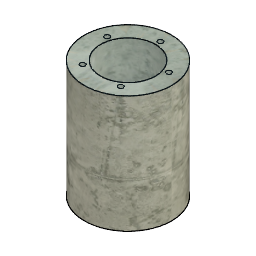
poken door (Autodesk Fusion 360 design; units mm, degrees)
Autodesk Fusion 360 part; units mm, degrees
note: some values were not read from the file. Chosen so that the rebuilt part matches the saved one: where a step ends.
sketch "Esboço1" plane through (0, 0, 0) normal (0, 0, 1) x (1, 0, 0)
  circle A0 centre (0, 0) radius 150
  dimension "d1" = 300
  constraint coincident A0.centre origin
  measures "d1" diameter of A0
extrude "Extrusão1" add sketch "Esboço1" along normal blind 470
sketch "Esboço2" plane through (0, 0, 470) normal (0, 0, 1) x (-1, 0, 0)
  circle A0 centre (0, 0) radius 150
  circle A1 centre (0, 0) radius 175
  dimension "d4" = 350
  constraint coincident A0.centre A1.centre
  measures "d4" diameter of A1
sketch "Esboço3" plane through (0, 0, 470) normal (0, 0, 1) x (-1, 0, 0)
extrude "Extrusão2" add sketch "Esboço2" along normal blind 0 and the other way blind 470
sketch "Esboço4" plane through (0, 0, 470) normal (0, 0, 1) x (-1, 0, 0)
  circle A0 centre (0, 0) radius 175
  circle A1 centre (0, 0) radius 150
  dimension "d10" = 300
  constraint concentric A0 A1
  measures "d10" diameter of A1
sketch "Esboço5" plane through (0, 0, 470) normal (0, 0, 1) x (-1, 0, 0)
  circle A0 centre (0, 0) radius 15
  dimension "d12" = 30
  constraint coincident A0.centre origin
  measures "d12" diameter of A0
ref_plane "Plano de trabalho2" through (0, 0, 370) normal (0, 0, 1) x (1, 0, 0)
sketch "Esboço10" plane through (0, 0, 0) normal (0, 0, -1) x (1, 0, 0)
  circle A0 centre (0, 0) radius 175
  circle A1 centre (0, 0) radius 110
  dimension "d22" = 220
  constraint coincident A0.centre A1.centre
  measures "d22" diameter of A1
sketch "Esboço11" plane through (0, 0, 0) normal (0, 0, -1) x (1, 0, 0)
  circle A0 centre (0, 0) radius 180
  dimension "d23" = 360
  constraint coincident A0.centre origin
  measures "d23" diameter of A0
extrude "Extrusão4" add sketch "Esboço11" along normal up to far side of body 1
sketch "Esboço14" plane through (0, 0, 470) normal (0, 0, 1) x (-1, 0, 0)
  circle A0 centre (0, 0) radius 175
  circle A1 centre (0, 0) radius 110
  dimension "d31" = 220
  constraint concentric A0 A1
  measures "d31" diameter of A1
extrude "Extrusão6" cut sketch "Esboço14" against normal through all contours A1
sketch "Esboço15" plane through (0, 0, 470) normal (0, 0, 1) x (-1, 0, 0)
  circle A0 centre (0, 0) radius 110
  circle A1 centre (0, 0) radius 175
  line L0 (0, 0) -> (0, -130)
  circle A2 centre (0, -130) radius 10
  circle A3 centre (123.6373, -40.1722) radius 10
  circle A4 centre (76.4121, 105.1722) radius 10
  circle A5 centre (-76.4121, 105.1722) radius 10
  circle A6 centre (-123.6373, -40.1722) radius 10
  dimension "d33" = 20
  dimension "d35" = 360
  dimension "d38" = 130
  constraint coincident A0.centre A1.centre
  constraint vertical L0
  constraint coincident L0.end A2.centre
  measures "d33" diameter of A2
  measures "d38" distance of A0.centre L0.end
extrude "Extrusão7" cut sketch "Esboço15" against normal blind 20 contours A2 | A3 | A4 | A5 | A6
sketch "Sketch18" plane through (0, 0, 470) normal (0, 0, 1) x (-1, 0, 0)
  circle A0 centre (0, 0) radius 175
  circle A1 centre (0, 0) radius 110
  circle A2 centre (123.6373, -40.1722) radius 10
  circle A3 centre (0, -130) radius 10
  circle A4 centre (76.4121, 105.1722) radius 10
  circle A5 centre (-123.6373, -40.1722) radius 10
  circle A6 centre (-76.4121, 105.1722) radius 10
